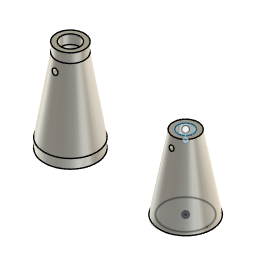
bocal secador v4 (Autodesk Fusion 360 design; units mm, degrees)
Autodesk Fusion 360 part; units mm, degrees
sketch "Esboço1" plane through (0, 0, 0) normal (0, 0, 1) x (1, 0, 0)
  circle A0 centre (0, 0) radius 23.1
  dimension "d1" = 46.2
  constraint coincident A0.centre origin
  measures "d1" diameter of A0
sketch "Esboço2" plane through (0, 0, 0) normal (0, 0, 1) x (1, 0, 0)
sketch "Esboço3" plane through (0, 0, 0) normal (0, 0, 1) x (1, 0, 0)
  circle A0 through (8.4, 0, 80) (-4.2, 7.2746, 80) (-4.2, -7.2746, 80)
  dimension "d2" = 16.8
loft "Transição1" add profiles "Esboço1", "Esboço3" section 1 section 2 contours A0 in plane through (0, 0, 80) normal (0, 0, 1) makes body 1
shell "Casca3" thickness 5 outward yes removed faces 2 at (-2.0838, 2.3218, 80) at (1.293, 6.4357, 0) on bodies 1
sketch "Esboço5" plane through (0, 0, 0) normal (0, 1, 0) x (1, 0, 0)
  circle A0 centre (0, -70) radius 2.5
  dimension "d11" = 5
  measures "d11" diameter of A0
extrude "Extrusão3" cut sketch "Esboço5" against normal blind 25 bodies 1
sketch "Esboço6" plane through (0, 0, 0) normal (0, 0, 1) x (1, 0, 0)
  circle A0 centre (-125, 0) radius 23.1
  circle A1 through (-114.9, 0, 80) (-130.05, 8.7469, 80) (-130.05, -8.7469, 80)
  dimension "d14" = 46.2
  dimension "d15" = 20.2
  measures "d14" diameter of A0
sketch "Esboço7" plane through (0, 0, 0) normal (0, 1, 0) x (1, 0, 0)
  circle A0 centre (-125, -70) radius 3
  dimension "d16" = 6
  measures "d16" diameter of A0
loft "Transição2" add profiles "Esboço6", "Esboço6" section 1 section 2 contours A1 in plane through (0, 0, 80) normal (0, 0, 1) separate body makes body 2
shell "Casca4" thickness 5 outward yes removed faces 2 at (-123.1328, -3.384, 80) at (-120.8939, 5.2713, 0) on bodies 2
extrude "Extrusão4" add 1 faces at (-111.617, -1.2552, 80) along direction (0, 0, 1) blind 10 on bodies 2 bodies 2
extrude "Extrusão5" add 1 faces at (-98.6278, -1.3993, 0) along direction (0, 0, -1) blind 10 on bodies 2 bodies 2
extrude "Extrusão6" cut sketch "Esboço7" against normal blind 25 bodies 2
move_body "Mover1" bodies 2 to x (1, 0, 0) y (0, 1, 0) z (0, 0, 1) at (0, 0, 10)
shell "Casca1" [suppressed]
delete_face "DeleteFace1" [suppressed]
sketch "Esboço4" plane through (0, 0, 0) normal (0, 1, 0) x (1, 0, 0)
  circle A0 through (2.3258, -68.5893, 13) (-1.5742, -66.3377, 13) (-1.5742, -70.841, 13)
  dimension "d4" = 5.2
extrude "Extrusão2" [suppressed]
shell "Casca2" [suppressed]
extrude "Extrusão1" [suppressed]
